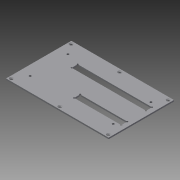
# Autodesk Inventor part: Driver4BusV11TopCorrected
Saved by Autodesk Inventor 2013 (Build 170138000, 138)
## iProperties
Created: 2014-07-28
Part Number: Driver4BusV11TopCorrected
Material: Generic
Document SubType Name: Sheet Metal
Designer: gsivil
Density: 1 g/cm^3
Sheet Metal Rule: Default
Author: gsivil
Autodesk Inventor part; units mm, degrees
ref_plane "YZ Plane" through (0, 0, 0) normal (1, 0, 0) x (0, 1, 0)
ref_plane "XZ Plane" through (0, 0, 0) normal (0, 1, 0) x (-1, 0, 0)
ref_plane "XY Plane" through (0, 0, 0) normal (0, 0, 1) x (1, 0, 0)
sketch "Sketch1" plane through (0, 0, 0) normal (0, 0, 1) x (1, 0, 0)
  line L0 (93.85, -64.2699) -> (-93.85, -64.2699)
  line L1 (-93.85, -64.2699) -> (-93.85, 55.2301)
  line L2 (-93.85, 55.2301) -> (93.85, 55.2301)
  line L3 (93.85, 55.2301) -> (93.85, -64.2699)
  line L4 (93.85, -64.2699) -> (-93.85, 55.2301) construction
  line L5 (-93.85, -64.2699) -> (93.85, 55.2301) construction
  point P0 (0, 0)
  point P1 (0, -4.5199)
  dimension "d0" = 187.7
  dimension "d1" = 119.5
  constraints: 12 end point, 2 midpoint, 2 parallel, 1 horizontal, 1 perpendicular
  measures "d0" distance of L1.end L2.end
  measures "d1" distance of L0.end L1.end
extrude "Extrusion1" add sketch "Sketch1" along normal mid plane 2.5
hole "Hole2" at (-88.85, -59.3199, 1.25) direction (0, 0, -1) diameter 4 end through all countersink diameter 7 countersink angle 90
hole "Hole3" at (0, -59.2699, 1.25) direction (0, 0, -1) diameter 4 end through all countersink diameter 7 countersink angle 90
hole "Hole4" at (88.9, -59.2699, 1.25) direction (0, 0, -1) diameter 4 end through all countersink diameter 7 countersink angle 90
hole "Hole5" at (-88.9, 50.2301, 1.25) direction (0, 0, -1) diameter 4 end through all countersink diameter 7 countersink angle 90
hole "Hole6" at (0, 50.2301, 1.25) direction (0, 0, -1) diameter 4 end through all countersink diameter 7 countersink angle 90
hole "Hole7" at (88.9, 50.2301, 1.25) direction (0, 0, -1) diameter 4 end through all countersink diameter 7 countersink angle 90
hole "Hole8" at (76.35, -38.2699, 1.25) direction (0, 0, -1) diameter 4 end through all
hole "Hole9" at (76.35, 30.7301, 1.25) direction (0, 0, -1) diameter 4 end through all
hole "Hole10" at (-75.65, -38.2699, 1.25) direction (0, 0, -1) diameter 4 end through all
hole "Hole11" at (-75.65, 30.7301, 1.25) direction (0, 0, -1) diameter 4 end through all
sketch "Sketch5" plane through (0, 0, 1.25) normal (0, 0, 1) x (1, 0, 0)
  circle A0 centre (76.35, -38.2699) radius 2 projected
  line L0 (93.85, -64.2699) -> (93.85, 55.2301) projected
  line L1 (-0.65, -21.7699) -> (85.35, -21.7699)
  line L2 (85.35, -21.7699) -> (85.35, -32.7699)
  line L3 (85.35, -32.7699) -> (-0.65, -32.7699)
  line L4 (-0.65, -32.7699) -> (-0.65, -21.7699)
  point P0 (0, 0)
  dimension "d120" = 8.5
  dimension "d121" = 5.5
  dimension "d122" = 11
  dimension "d123" = 86
  constraints: 8 end point, 2 parallel, 1 horizontal, 1 perpendicular
  measures "d120" distance between parallel lines of L0 L2
  measures "d121" distance from line of A0.centre L3
  measures "d122" distance between parallel lines of L1 L3
  measures "d123" distance between parallel lines of L4 L2
extrude "Cut1" cut sketch "Sketch5" along normal through all both and the other way through all contours L1 L2 L3 L4
pattern_linear "Rectangular Pattern1" count 2 spacing 45.5 along (0, 1, 0) of "Cut1"
hole "Hole19" at (85.35, 12.7301, 1.25) direction (0, 0, -1) diameter 3 end through all
hole "Hole20" at (85.35, 23.7301, 1.25) direction (0, 0, -1) diameter 3 end through all
hole "Hole23" at (85.35, -21.7699, 1.25) direction (0, 0, -1) diameter 3 end through all
hole "Hole24" at (85.35, -32.7699, 1.25) direction (0, 0, -1) diameter 3 end through all
sketch "Sketch8" plane through (0, 0, 1.25) normal (0, 0, 1) x (1, 0, 0)
  arc A0 (-0.65, 14.2301) -> (0.85, 12.7301) centre (-0.65, 12.7301) ccw projected
  line L0 (-0.65, 12.7301) -> (-0.65, 23.7301) projected
  arc A1 (0.85, 23.7301) -> (-0.65, 22.2301) centre (-0.65, 23.7301) ccw projected
  line L1 (-0.65, 23.7301) -> (-0.65, 12.7301)
  line L2 (-0.65, 12.7301) -> (-50.65, 12.7301)
  line L3 (-50.65, 12.7301) -> (-50.65, 23.7301)
  line L4 (-50.65, 23.7301) -> (-0.65, 23.7301)
  arc A2 (83.85, -32.7699) -> (85.35, -31.2699) centre (85.35, -32.7699) ccw projected
  line L5 (83.85, -32.7699) -> (-0.65, -32.7699) projected
  line L6 (-0.65, -32.7699) -> (-0.65, -21.7699) projected
  line L7 (-0.65, -21.7699) -> (83.85, -21.7699) projected
  arc A3 (85.35, -23.2699) -> (83.85, -21.7699) centre (85.35, -21.7699) ccw projected
  line L8 (85.35, -23.2699) -> (85.35, -31.2699) projected
  arc A4 (85.35, 22.2301) -> (83.85, 23.7301) centre (85.35, 23.7301) ccw projected
  line L9 (85.35, 22.2301) -> (85.35, 14.2301) projected
  arc A5 (83.85, 12.7301) -> (85.35, 14.2301) centre (85.35, 12.7301) ccw projected
  line L10 (83.85, 12.7301) -> (-0.65, 12.7301) projected
  line L11 (-0.65, 12.7301) -> (-0.65, 23.7301) projected
  line L12 (-0.65, 23.7301) -> (83.85, 23.7301) projected
  circle A6 centre (-75.65, 30.7301) radius 2 projected
  circle A7 centre (-75.65, -38.2699) radius 2 projected
  circle A8 centre (76.35, 30.7301) radius 2 projected
  circle A9 centre (76.35, -38.2699) radius 2 projected
  circle A10 centre (88.9, 50.2301) radius 3.5 projected
  circle A11 centre (0, 50.2301) radius 3.5 projected
  circle A12 centre (-88.9, 50.2301) radius 3.5 projected
  circle A13 centre (88.9, -59.2699) radius 3.5 projected
  circle A14 centre (0, -59.2699) radius 3.5 projected
  circle A15 centre (-88.85, -59.3199) radius 3.5 projected
  line L13 (-93.85, -64.2699) -> (93.85, -64.2699) projected
  line L14 (93.85, -64.2699) -> (93.85, 55.2301) projected
  line L15 (93.85, 55.2301) -> (-93.85, 55.2301) projected
  line L16 (-93.85, 55.2301) -> (-93.85, -64.2699) projected
  point P0 (0, 0)
  dimension "d273" = 50
  constraints: 8 end point, 3 equal length, 1 perpendicular
  measures "d273" distance of L0.start L2.end
extrude "Cut4" cut sketch "Sketch8" against normal through all contours L0 L2 A0 | A0 L2 L3 L4 A1 L0 | A1 L4 L0
hole "Hole27" at (-50.65, 23.7301, 1.25) direction (0, 0, -1) diameter 3 end through all
hole "Hole28" at (-50.65, 12.7301, 1.25) direction (0, 0, -1) diameter 3 end through all
hole "Hole29" at (-0.65, -21.7699, 1.25) direction (0, 0, -1) diameter 3 end through all
hole "Hole30" at (-0.65, -32.7699, 1.25) direction (0, 0, -1) diameter 3 end through all
equation "\"d124\" = Thickness"
equation "\"d205\" = Thickness"
equation "\"d214\" = Thickness"
equation "\"d241\" = Thickness"
equation "\"d250\" = Thickness"
equation "\"d274\" = Thickness"
equation "\"d283\" = Thickness"
equation "\"d292\" = Thickness"
equation "\"d301\" = Thickness"
equation "\"d310\" = Thickness"
equation "\"BendRadius\" = Thickness"
equation "\"BendReliefWidth\" = Thickness"
equation "\"BendReliefDepth\" = 0.5 * Thickness"
equation "\"CornerReliefSize\" = 4 * Thickness"
equation "\"MinimumRemnant\" = 2 * Thickness"
equation "\"TransitionRadius\" = BendRadius"
equation "\"JacobiRadiusSize\" = Thickness"
equation "\"GapSize\" = Thickness"
equation "\"Thickness\" = 0.5"
body "Solid1"
